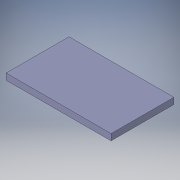
# Autodesk Inventor part: stamp5x3
Saved by Autodesk Inventor 2019 (Build 230136000, 136)
## iProperties
Created: 2019-02-19
Part Number: stamp5x3
Material: PET Plastic
Document SubType Name: Modeling
Designer: jmc
Density: 1.541 g/cm^3
Appearance: Slate Blue
Author: jmc
Autodesk Inventor part; units mm, degrees
ref_plane "YZ Plane" through (0, 0, 0) normal (1, 0, 0) x (0, 1, 0)
ref_plane "XZ Plane" through (0, 0, 0) normal (0, 1, 0) x (-1, 0, 0)
ref_plane "XY Plane" through (0, 0, 0) normal (0, 0, 1) x (1, 0, 0)
sketch "Sketch1" plane through (0, 0, 0) normal (0, 1, 0) x (-1, 0, 0)
  line L0 (24.925, 14.925) -> (-24.925, 14.925)
  line L1 (-24.925, 14.925) -> (-24.925, -14.925)
  line L2 (-24.925, -14.925) -> (24.925, -14.925)
  line L3 (24.925, 14.925) -> (-24.925, -14.925) construction
  line L4 (-24.925, 14.925) -> (24.925, -14.925) construction
  line L5 (24.925, -14.925) -> (24.925, 14.925)
  line L6 (24.925, 5) -> (24.925, 14.925)
  point P0 (0, 0)
  dimension "d0" = 49.85
  dimension "d1" = 29.85
  constraints: 14 end point, 3 parallel, 2 midpoint, 1 horizontal, 1 perpendicular
  measures "d0" distance of L2.end L1.end
  measures "d1" distance of L1.end L0.end
extrude "Extrusion1" add sketch "Sketch1" along normal blind 3
sketch "Sketch2" plane through (0, 0, 0) normal (0, -1, 0) x (1, 0, 0)
  point P0 (0, 0)
sketch "Sketch3" plane through (-24.925, 0, -14.925) normal (-1, 0, 0) x (0, 0, 1)
  point P0 (14.925, 0)
sketch "Sketch4" plane through (0, 0, 0) normal (0, -1, 0) x (1, 0, 0)
  line L0 (-24.925, 14.925) -> (-24.925, -14.925) construction
  line L1 (-18.0744, 9.3011) -> (17.0849, 9.3011) construction
  line L2 (17.0849, 9.3011) -> (17.0849, -10.8842) construction
  line L3 (17.0849, -10.8842) -> (-18.0744, -10.8842) construction
  line L4 (-18.0744, -10.8842) -> (-18.0744, 9.3011) construction
  line L5 (-11.4806, 4.7344) -> (-14.0804, 4.7344)
  line L6 (-14.0804, 4.7344) -> (-14.0804, 6.4751)
  spline S0 degree 2 poles (-14.0804, 6.4751) (-14.0804, 7.2287) (-14.2462, 7.6055) (-14.5326, 7.6055) knots 0 0 0 1 2 2 2
  spline S1 degree 2 poles (-14.5326, 7.6055) (-14.8566, 7.6055) (-15.03, 7.1458) (-15.03, 6.3923) knots 0 0 0 1 2 2 2
  line L7 (-15.03, 6.3923) -> (-15.03, 1.7502)
  spline S2 degree 2 poles (-15.03, 1.7502) (-15.03, 1.0192) (-14.8566, 0.5746) (-14.5552, 0.5746) knots 0 0 0 1 2 2 2
  spline S3 degree 2 poles (-14.5552, 0.5746) (-14.2613, 0.5746) (-14.0804, 1.0192) (-14.0804, 1.8406) knots 0 0 0 1 2 2 2
  line L8 (-14.0804, 1.8406) -> (-14.0804, 3.0991)
  line L9 (-14.0804, 3.0991) -> (-11.4806, 3.0991)
  line L10 (-11.4806, 3.0991) -> (-11.4806, 2.7072)
  spline S4 degree 2 poles (-11.4806, 2.7072) (-11.4806, 1.1549) (-11.9177, -0.1413) (-13.4248, -1.1209) (-14.5175, -1.1209) knots 0 0 0 1 2 3 3 3
  spline S5 degree 2 poles (-14.5175, -1.1209) (-15.663, -1.1209) (-17.1475, -0.292) (-17.6298, 1.1699) (-17.6298, 2.6394) knots 0 0 0 1 2 3 3 3
  line L11 (-17.6298, 2.6394) -> (-17.6298, 5.5633)
  spline S6 degree 2 poles (-17.6298, 5.5633) (-17.6298, 6.6409) (-17.4791, 7.7261) (-16.7481, 8.7283) (-15.4444, 9.3011) (-14.5929, 9.3011) knots 0 0 0 1 2 3 4 4 4
  spline S7 degree 2 poles (-14.5929, 9.3011) (-13.4474, 9.3011) (-11.9478, 8.4118) (-11.4806, 7.0855) (-11.4806, 5.6839) knots 0 0 0 1 2 3 3 3
  line L12 (-11.4806, 5.6839) -> (-11.4806, 4.7344)
  line L13 (-10.5462, 9.0901) -> (-8.7074, 9.0901)
  spline S8 degree 2 poles (-8.7074, 9.0901) (-6.8687, 9.0901) (-5.565, 8.8037) (-4.7436, 7.6357) (-4.7436, 6.3621) knots 0 0 0 1 2 3 3 3
  spline S9 degree 2 poles (-4.7436, 6.3621) (-4.7436, 5.1941) (-5.3238, 4.3877) (-6.1754, 4.3048) knots 0 0 0 1 2 2 2
  spline S10 degree 2 poles (-6.1754, 4.3048) (-5.4067, 4.1164) (-4.8717, 3.4759) (-4.7436, 2.9409) (-4.7436, 1.7276) knots 0 0 0 1 2 3 3 3
  line L14 (-4.7436, 1.7276) -> (-4.7436, -0.9099)
  line L15 (-4.7436, -0.9099) -> (-7.1626, -0.9099)
  line L16 (-7.1626, -0.9099) -> (-7.1626, 2.4134)
  spline S11 degree 2 poles (-7.1626, 2.4134) (-7.1626, 3.2121) (-7.4113, 3.5965) (-7.9463, 3.5965) knots 0 0 0 1 2 2 2
  line L17 (-7.9463, 3.5965) -> (-7.9463, -0.9099)
  line L18 (-7.9463, -0.9099) -> (-10.5462, -0.9099)
  line L19 (-10.5462, -0.9099) -> (-10.5462, 9.0901)
  line L20 (-7.9463, 7.3794) -> (-7.9463, 5.1564)
  spline S12 degree 2 poles (-7.9463, 5.1564) (-7.5092, 5.1564) (-7.1626, 5.3975) (-7.1626, 6.0607) knots 0 0 0 1 2 2 2
  line L21 (-7.1626, 6.0607) -> (-7.1626, 6.6108)
  spline S13 degree 2 poles (-7.1626, 6.6108) (-7.1626, 7.0855) (-7.5017, 7.3794) (-7.9463, 7.3794) knots 0 0 0 1 2 2 2
  line L22 (0.7575, 9.0901) -> (2.2496, -0.9099)
  line L23 (2.2496, -0.9099) -> (-0.418, -0.9099)
  line L24 (-0.418, -0.9099) -> (-0.5537, 0.8911)
  line L25 (-0.5537, 0.8911) -> (-1.4806, 0.8911)
  line L26 (-1.4806, 0.8911) -> (-1.6313, -0.9099)
  line L27 (-1.6313, -0.9099) -> (-4.3291, -0.9099)
  line L28 (-4.3291, -0.9099) -> (-3.0104, 9.0901)
  line L29 (-3.0104, 9.0901) -> (0.7575, 9.0901)
  spline S14 degree 2 poles (-0.6215, 2.662) (-0.8099, 4.3576) (-1.0134, 6.8595) knots 0 0 0 1 1 1
  spline S15 degree 2 poles (-1.0134, 6.8595) (-1.4052, 3.9883) (-1.5107, 2.662) knots 0 0 0 1 1 1
  line L30 (-1.5107, 2.662) -> (-0.6215, 2.662)
  line L31 (2.6942, 9.0901) -> (5.3167, 9.0901)
  spline S16 degree 2 poles (5.3167, 9.0901) (6.3792, 9.0901) (7.5247, 8.7585) (8.0974, 8.1255) (8.3009, 7.2287) (8.3009, 6.2943) knots 0 0 0 1 2 3 4 4 4
  line L32 (8.3009, 6.2943) -> (8.3009, 5.4201)
  spline S17 degree 2 poles (8.3009, 5.4201) (8.3009, 4.4631) (7.9015, 3.5814) (6.8465, 3.1142) (5.9949, 3.1142) knots 0 0 0 1 2 3 3 3
  line L33 (5.9949, 3.1142) -> (5.2941, 3.1142)
  line L34 (5.2941, 3.1142) -> (5.2941, -0.9099)
  line L35 (5.2941, -0.9099) -> (2.6942, -0.9099)
  line L36 (2.6942, -0.9099) -> (2.6942, 9.0901)
  line L37 (5.2941, 7.3794) -> (5.2941, 4.8323)
  spline S18 degree 2 poles (5.2941, 4.8323) (5.4071, 4.8248) (5.4825, 4.8248) knots 0 0 0 1 1 1
  spline S19 degree 2 poles (5.4825, 4.8248) (5.8442, 4.8248) (6.123, 5.179) (6.123, 5.7366) knots 0 0 0 1 2 2 2
  line L38 (6.123, 5.7366) -> (6.123, 6.558)
  spline S20 degree 2 poles (6.123, 6.558) (6.123, 7.0705) (5.799, 7.3794) (5.2941, 7.3794) knots 0 0 0 1 2 2 2
  point P0 (0, 0)
  constraints: 2 other
extrude "Extrusion2" add sketch "Sketch4" along normal blind 1
body "Solid1"
